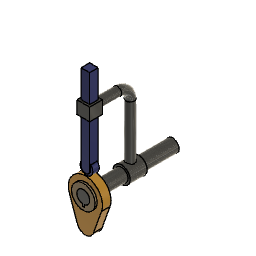
Cam Follower v2 (Autodesk Fusion 360 design; units mm, degrees)
Autodesk Fusion 360 part; units mm, degrees
note: some values were not read from the file. Set by a fixed rule: which sketch regions a step uses.
sketch "Sketch1" plane through (0, 0, 0) normal (0, 1, 0) x (1, 0, 0) in component "Cam"
  circle A0 centre (0, 0) radius 27.5
  circle A1 centre (0, 0) radius 40
  circle A2 centre (0, 60) radius 20
  line L0 (-37.7124, 13.3333) -> (-18.8562, 66.6667)
  line L1 (18.8562, 66.6667) -> (37.7124, 13.3333)
  line L2 (-2.5, 14.7902) -> (-2.5, 20)
  line L3 (-2.5, 20) -> (2.5, 20)
  line L4 (2.5, 20) -> (2.5, 14.7902)
  arc A3 (-2.5, 14.7902) -> (2.5, 14.7902) centre (0, 0) ccw
  dimension "d1" = 30
  dimension "d2" = 55
  dimension "d3" = 80
  dimension "d4" = 40
  dimension "d5" = 60
  dimension "d6" = 5
  constraint coincident A0.centre A1.centre
  constraint concentric A0 A3
  constraint coincident A1 L0.start
  constraint coincident A2 L0.end
  constraint tangent A2 L0
  constraint coincident A2 L1.start
  constraint coincident A1 L1.end
  constraint tangent A1 L1
  constraint tangent A1 L0
  constraint tangent A2 L1
  constraint parallel L2 L4
  measures "d1" diameter of A3
  measures "d2" diameter of A0
  measures "d3" diameter of A1
  measures "d4" diameter of A2
  measures "d5" distance of A0.centre A2.centre
  measures "d6" distance of L2.end L3.end
extrude "Extrude1" add sketch "Sketch1" along normal mid plane 20 contours A1 | A1 A2 L1 | A1 A2 L0 | A2 makes body 1 in component "Cam"
extrude "Extrude2" add sketch "Sketch1" along normal mid plane 30 separate body contours A0 makes body 2 in component "Cam"
sketch "Sketch1 (2)" plane through (0, 0, 0) normal (0, 1, 0) x (1, 0, 0) in component "Follower"
  circle A0 centre (0, -55) radius 15
  line L0 (10, -55) -> (10, -255)
  line L1 (10, -255) -> (-10, -255)
  line L2 (-10, -255) -> (-10, -55)
  arc A1 (10, -55) -> (-10, -55) centre (0, -55) ccw
  dimension "d12" = 30
  dimension "d13" = 20
  dimension "d14" = 20
  dimension "d15" = 200
  constraint concentric A0 A1
  constraint vertical L0
  constraint horizontal L1
  constraint vertical L2
  measures "d12" diameter of A0
  measures "d13" diameter of A1
  measures "d14" distance of L2.end L0.start
  measures "d15" distance of L2.end L1.end
extrude "Extrude1'" add sketch "Sketch1 (2)" along normal mid plane 15 separate body contours A0 L0 L2 A1 | A0 L0 L2 A1 makes body 3 in component "Follower"
extrude "Extrude2'" add sketch "Sketch1 (2)" along normal mid plane 20 separate body contours A0 L0 L2 A1 | A0 L0 L1 L2 picked at (0, -60) makes body 4 in component "Follower"
combine "Combine1" operation cut target body 4 tool bodies 3 keep tools in component "Follower"
sketch "Sketch1 (3)" plane through (0, 0, 0) normal (0, 1, 0) x (1, 0, 0) in component "Shafft"
  line L0 (-2.5, 20) -> (-2.5, 14.7902)
  arc A0 (-2.5, 14.7902) -> (2.5, 14.7902) centre (0, 0) ccw
  line L1 (2.5, 14.7902) -> (2.5, 20)
  line L2 (2.5, 20) -> (-2.5, 20)
  circle A1 centre (0, 0) radius 27.5
extrude "Extrude1''" add sketch "Sketch1 (3)" along normal mid plane 30 separate body contours L0 A0 L1 L2 makes body 5 in component "Shafft"
cylinder "CylinderPrimitive1" add diameter 30 height 180 placed x (1, 0, 0) y (0, 0, -1) z (0, 1, 0) at (0, 15, 0) bodies 5 in component "Shafft"
sketch "Sketch1 (4)" plane through (0, 0, 0) normal (1, 0, 0) x (0, 1, 0) in component "Base"
  line L0 (195, -15) -> (195, 15)
  line L1 (-15, 15) -> (-15, -14.7902)
  line L2 (-15, -14.7902) -> (-15, -20)
  line L3 (15, -20) -> (15, -15)
  line L4 (-15, -20) -> (15, -20)
  line L5 (15, -15) -> (195, -15)
  line L6 (-15, 15) -> (195, 15)
  line L7 (75, 15) -> (115, 15)
  line L8 (115, 15) -> (115, 20)
  line L9 (115, 20) -> (75, 20)
  line L10 (75, 20) -> (75, 15)
  line L11 (15, -27.5) -> (15, 27.5)
  line L12 (95, 15) -> (95, 145)
  line L13 (65, 175) -> (15, 175)
  arc A0 (95, 145) -> (65, 175) centre (65, 145) ccw
  point P0 (95, 175)
  dimension "d24" = 40
  dimension "d25" = 5
  dimension "d26" = 60
  dimension "d27" = 160
  dimension "d28" = 80
  dimension "d29" = 30
  constraint horizontal L7
  constraint vertical L8
  constraint horizontal L9
  constraint vertical L10
  constraint coincident L6 L7.start
  constraint midpoint L7 L12.start
  constraint perpendicular L7 L12
  constraint perpendicular L12 L13
  constraint coincident P0 L12
  constraint coincident P0 L13
  constraint tangent L12 A0
  constraint tangent L13 A0
  measures "d24" distance of L7.start L7.end
  measures "d25" distance of L7.start L9.end
  measures "d26" distance of L7.start L11
  measures "d27" distance of L12.start P0
  measures "d28" distance of P0 L13.end
  measures "d29" radius of A0
revolve "Revolve1" add sketch "Sketch1 (4)" angle 360 about axis through (0, 0, 0) along (0, -1, 0) separate body contours L6 L7 L8 L9 L12 | L6 L7 L9 L10 L12 makes body 6 in component "Base"
pipe "Pipe1" add diameter 20 path "Sketch1 (4)" along L13 A0 L12 separate body makes body 7
ref_plane "WorkPlane1" through (0, 40, 175) normal (0, 0, 1) x (0, -1, 0)
sketch "Sketch1 (5)" plane through (0, 40, 175) normal (0, 0, 1) x (1, 0, 0)
  line L0 (10, -47.5) -> (10, -32.5)
  line L1 (-10, -32.5) -> (-10, -47.5)
  line L2 (-10, -50) -> (-10, -47.5)
  line L3 (-10, -32.5) -> (-10, -30)
  line L4 (10, -50) -> (10, -47.5)
  line L5 (-10, -50) -> (10, -50)
  line L6 (10, -30) -> (-10, -30)
  line L7 (10, -32.5) -> (10, -30)
  line L8 (10, -30) -> (-10, -30)
  line L9 (-10, -30) -> (-10, -50)
  line L10 (-10, -50) -> (10, -50)
  line L11 (10, -50) -> (10, -30)
  line L12 (10, -30) -> (-10, -50) construction
  line L13 (-10, -30) -> (10, -50) construction
  line L14 (-15, -25) -> (-15, -55)
  line L15 (-15, -55) -> (15, -55)
  line L16 (15, -55) -> (15, -25)
  line L17 (15, -25) -> (-15, -25)
  point P0 (0, -40)
  dimension "d36" = 5
  constraint horizontal L8
  constraint perpendicular L8 L9
  constraint parallel L8 L10
  constraint parallel L9 L11
  constraint coincident L12 P0
  constraint coincident L13 P0
  constraint coincident L6.start L7.end
extrude "Extrude1'''" add sketch "Sketch1 (5)" along normal mid plane 30 bodies 7
copy_body "CutPasteBodies1" bodies 7 removing the originals makes body 8 in component "Base"
combine "Combine1'" operation add target body 8 tool bodies 6 keep tools in component "Base"
combine "Combine2" operation cut target body 4 tool bodies 8 keep tools in component "Follower"
combine "Combine2'" operation cut target body 8 tool bodies 5 keep tools in component "Base"
component "Cam" placed x (1, 0, 0) y (0, 1, 0) z (0, 0, 1) at (0, 0, 0)
component "Follower" placed x (1, 0, 0) y (0, 1, 0) z (0, 0, 1) at (0, 0, 0)
component "Shafft" placed x (1, 0, 0) y (0, 1, 0) z (0, 0, 1) at (0, 0, 0)
component "Base" placed x (1, 0, 0) y (0, 1, 0) z (0, 0, 1) at (0, 0, 0)
